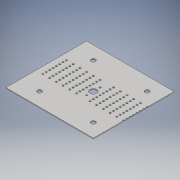
# Autodesk Inventor part: Drill Jig Base
Saved by Autodesk Inventor 2018 (Build 220112000, 112)
## iProperties
Created: 2018-12-05
Part Number: Drill Jig Base
Material: Generic
Document SubType Name: Modeling
Designer: gbgic
Density: 1 g/cm^3
Appearance: Default
Author: gbgic
Autodesk Inventor part; units mm, degrees
ref_plane "YZ Plane" through (0, 0, 0) normal (1, 0, 0) x (0, 1, 0)
ref_plane "XZ Plane" through (0, 0, 0) normal (0, 1, 0) x (-1, 0, 0)
ref_plane "XY Plane" through (0, 0, 0) normal (0, 0, 1) x (1, 0, 0)
sketch "Sketch1" plane through (0, 0, 0) normal (1, 0, 0) x (0, 1, 0)
  line L0 (4.9868, -9.3187) -> (4.9868, 295.4813)
  line L1 (4.9868, 295.4813) -> (-325.2132, 295.4813)
  line L2 (4.9868, -9.3187) -> (-325.2132, -9.3187)
  line L3 (-325.2132, 295.4813) -> (-325.2132, -9.3187)
  point P0 (0, 0)
  dimension "d73" = 330.2
  dimension "d74" = 330.2
  dimension "d75" = 304.8
  constraints: 8 end point, 2 horizontal, 1 vertical
  measures "d73" distance of L0.end L1.end
  measures "d74" distance of L0.start L2.end
  measures "d75" distance of L1.end L2.end
extrude "Extrusion1" add sketch "Sketch1" along normal blind 3.175
sketch "Sketch2" plane through (3.175, 0, 0) normal (1, 0, 0) x (0, 0, -1)
  line L0 (-143.0813, 4.9868) -> (-143.0813, -147.4132)
  circle A0 centre (-143.0813, -147.4132) radius 12.7
  point P0 (0, 0)
  point P1 (9.3187, 4.9868)
  dimension "d4" = 152.4
  dimension "d5" = 25.4
  constraints: 2 end point, 1 centre point, 1 coincident
  measures "d4" distance of L0.start L0.end
  measures "d5" diameter of A0
extrude "Extrusion2" cut sketch "Sketch2" against normal blind 50.8
sketch "Sketch3" plane through (3.175, 0, 0) normal (1, 0, 0) x (0, 0, -1)
  circle A0 centre (-143.0813, -147.4132) radius 12.7 projected
  circle A1 centre (-143.0813, -122.0132) radius 3.175
  circle A2 centre (-143.0813, -96.6132) radius 3.175
  circle A3 centre (-143.0813, -71.2132) radius 3.175
  circle A4 centre (-143.0813, -45.8132) radius 3.175
  circle A5 centre (-143.0813, -20.4132) radius 3.175
  circle A6 centre (-143.0813, 4.9868) radius 3.175
  line L0 (9.3187, -299.8132) -> (9.3187, 4.9868) projected
  circle A7 centre (-143.0813, -172.8132) radius 3.175
  circle A8 centre (-143.0813, -198.2132) radius 3.175
  circle A9 centre (-143.0813, -249.0132) radius 3.175
  circle A10 centre (-143.0813, -223.6132) radius 3.175
  circle A11 centre (-143.0813, -299.8132) radius 3.175
  circle A12 centre (-143.0813, -274.4132) radius 3.175
  circle A13 centre (-155.7813, -122.0132) radius 3.175
  circle A14 centre (-155.7813, -96.6132) radius 3.175
  circle A15 centre (-155.7813, -45.8132) radius 3.175
  circle A16 centre (-155.7813, -71.2132) radius 3.175
  circle A17 centre (-155.7813, 4.9868) radius 3.175
  circle A18 centre (-155.7813, -20.4132) radius 3.175
  circle A19 centre (-155.7813, -299.8132) radius 3.175
  circle A20 centre (-155.7813, -249.0132) radius 3.175
  circle A21 centre (-155.7813, -274.4132) radius 3.175
  circle A22 centre (-155.7813, -223.6132) radius 3.175
  circle A23 centre (-155.7813, -198.2132) radius 3.175
  circle A24 centre (-155.7813, -172.8132) radius 3.175
  line L1 (-155.7813, -299.8132) -> (-168.4813, -299.8132) construction
  line L2 (-168.4813, -299.8132) -> (-181.1813, -299.8132) construction
  line L3 (-181.1813, -299.8132) -> (-193.8813, -299.8132) construction
  line L4 (-143.0813, -299.8132) -> (-130.3813, -299.8132) construction
  line L5 (-130.3813, -299.8132) -> (-117.6813, -299.8132) construction
  line L6 (-117.6813, -299.8132) -> (-104.9813, -299.8132) construction
  circle A25 centre (-168.4813, -122.0132) radius 3.175
  circle A26 centre (-168.4813, -96.6132) radius 3.175
  circle A27 centre (-168.4813, -45.8132) radius 3.175
  circle A28 centre (-168.4813, -71.2132) radius 3.175
  circle A29 centre (-168.4813, 4.9868) radius 3.175
  circle A30 centre (-168.4813, -20.4132) radius 3.175
  circle A31 centre (-168.4813, -299.8132) radius 3.175
  circle A32 centre (-168.4813, -249.0132) radius 3.175
  circle A33 centre (-168.4813, -274.4132) radius 3.175
  circle A34 centre (-168.4813, -223.6132) radius 3.175
  circle A35 centre (-168.4813, -198.2132) radius 3.175
  circle A36 centre (-168.4813, -172.8132) radius 3.175
  circle A37 centre (-181.1813, -122.0132) radius 3.175
  circle A38 centre (-181.1813, -96.6132) radius 3.175
  circle A39 centre (-181.1813, -45.8132) radius 3.175
  circle A40 centre (-181.1813, -71.2132) radius 3.175
  circle A41 centre (-181.1813, 4.9868) radius 3.175
  circle A42 centre (-181.1813, -20.4132) radius 3.175
  circle A43 centre (-181.1813, -299.8132) radius 3.175
  circle A44 centre (-181.1813, -249.0132) radius 3.175
  circle A45 centre (-181.1813, -274.4132) radius 3.175
  circle A46 centre (-181.1813, -223.6132) radius 3.175
  circle A47 centre (-181.1813, -198.2132) radius 3.175
  circle A48 centre (-181.1813, -172.8132) radius 3.175
  circle A49 centre (-193.8813, -122.0132) radius 3.175
  circle A50 centre (-193.8813, -96.6132) radius 3.175
  circle A51 centre (-193.8813, -45.8132) radius 3.175
  circle A52 centre (-193.8813, -71.2132) radius 3.175
  circle A53 centre (-193.8813, 4.9868) radius 3.175
  circle A54 centre (-193.8813, -20.4132) radius 3.175
  circle A55 centre (-193.8813, -299.8132) radius 3.175
  circle A56 centre (-193.8813, -249.0132) radius 3.175
  circle A57 centre (-193.8813, -274.4132) radius 3.175
  circle A58 centre (-193.8813, -223.6132) radius 3.175
  circle A59 centre (-193.8813, -198.2132) radius 3.175
  circle A60 centre (-193.8813, -172.8132) radius 3.175
  circle A61 centre (-130.3813, -122.0132) radius 3.175
  circle A62 centre (-130.3813, -96.6132) radius 3.175
  circle A63 centre (-130.3813, -45.8132) radius 3.175
  circle A64 centre (-130.3813, -71.2132) radius 3.175
  circle A65 centre (-130.3813, 4.9868) radius 3.175
  circle A66 centre (-130.3813, -20.4132) radius 3.175
  circle A67 centre (-130.3813, -299.8132) radius 3.175
  circle A68 centre (-130.3813, -249.0132) radius 3.175
  circle A69 centre (-130.3813, -274.4132) radius 3.175
  circle A70 centre (-130.3813, -223.6132) radius 3.175
  circle A71 centre (-130.3813, -198.2132) radius 3.175
  circle A72 centre (-130.3813, -172.8132) radius 3.175
  line L7 (-117.6813, -299.8132) -> (-104.9813, -299.8132) construction
  circle A73 centre (-117.6813, -299.8132) radius 3.175
  circle A74 centre (-117.6813, -45.8132) radius 3.175
  circle A75 centre (-117.6813, -71.2132) radius 3.175
  circle A76 centre (-117.6813, -96.6132) radius 3.175
  circle A77 centre (-117.6813, -122.0132) radius 3.175
  circle A78 centre (-117.6813, 4.9868) radius 3.175
  circle A79 centre (-117.6813, -274.4132) radius 3.175
  circle A80 centre (-117.6813, -249.0132) radius 3.175
  circle A81 centre (-117.6813, -223.6132) radius 3.175
  circle A82 centre (-117.6813, -198.2132) radius 3.175
  circle A83 centre (-117.6813, -172.8132) radius 3.175
  circle A84 centre (-117.6813, -20.4132) radius 3.175
  line L8 (-104.9813, -299.8132) -> (-92.2813, -299.8132) construction
  circle A85 centre (-104.9813, -299.8132) radius 3.175
  circle A86 centre (-104.9813, -45.8132) radius 3.175
  circle A87 centre (-104.9813, -71.2132) radius 3.175
  circle A88 centre (-104.9813, -96.6132) radius 3.175
  circle A89 centre (-104.9813, -122.0132) radius 3.175
  circle A90 centre (-104.9813, 4.9868) radius 3.175
  circle A91 centre (-104.9813, -274.4132) radius 3.175
  circle A92 centre (-104.9813, -249.0132) radius 3.175
  circle A93 centre (-104.9813, -223.6132) radius 3.175
  circle A94 centre (-104.9813, -198.2132) radius 3.175
  circle A95 centre (-104.9813, -172.8132) radius 3.175
  circle A96 centre (-104.9813, -20.4132) radius 3.175
  point P0 (0, 0)
  dimension "d9" = 6.35
  dimension "d11" = 6.35
  dimension "d12" = 6.35
  dimension "d13" = 6.35
  dimension "d14" = 6.35
  dimension "d15" = 6.35
  dimension "d77" = 6.35
  dimension "d78" = 6.35
  dimension "d79" = 6.35
  dimension "d80" = 6.35
  dimension "d81" = 6.35
  dimension "d82" = 6.35
  dimension "d83" = 12.7
  dimension "d84" = 12.7
  dimension "d85" = 12.7
  dimension "d86" = 12.7
  dimension "d87" = 12.7
  dimension "d88" = 12.7
  dimension "d89" = 6.35
  dimension "d90" = 6.35
  dimension "d91" = 6.35
  dimension "d92" = 6.35
  dimension "d93" = 6.35
  dimension "d94" = 6.35
  dimension "d95" = 6.35
  dimension "d96" = 6.35
  dimension "d97" = 6.35
  dimension "d98" = 6.35
  dimension "d99" = 6.35
  dimension "d100" = 6.35
  dimension "d101" = 6.35
  dimension "d102" = 6.35
  dimension "d103" = 6.35
  dimension "d104" = 6.35
  dimension "d105" = 6.35
  dimension "d106" = 6.35
  dimension "d107" = 6.35
  dimension "d108" = 6.35
  dimension "d109" = 6.35
  dimension "d110" = 6.35
  dimension "d111" = 6.35
  dimension "d112" = 6.35
  dimension "d113" = 12.7
  dimension "d114" = 6.35
  dimension "d115" = 6.35
  dimension "d116" = 6.35
  dimension "d117" = 6.35
  dimension "d118" = 6.35
  dimension "d119" = 6.35
  dimension "d120" = 12.7
  dimension "d121" = 6.35
  dimension "d122" = 6.35
  dimension "d123" = 6.35
  dimension "d124" = 6.35
  dimension "d125" = 6.35
  dimension "d126" = 6.35
  constraints: 96 centre point, 16 end point, 5 horizontal, 3 point on line
  measures "d9" diameter of A1
  measures "d11" diameter of A2
  measures "d12" diameter of A3
  measures "d13" diameter of A4
  measures "d14" diameter of A5
  measures "d15" diameter of A6
  measures "d77" diameter of A13
  measures "d78" diameter of A14
  measures "d79" diameter of A16
  measures "d80" diameter of A15
  measures "d81" diameter of A18
  measures "d82" diameter of A17
  measures "d83" distance of L1.start L1.end
  measures "d84" distance of L1.end L2.end
  measures "d85" distance of L2.end L3.end
  measures "d86" distance of L4.start L4.end
  measures "d87" distance of L5.end L4.end
  measures "d88" distance of L5.end L6.end
  measures "d89" diameter of A25
  measures "d90" diameter of A26
  measures "d91" diameter of A28
  measures "d92" diameter of A27
  measures "d93" diameter of A30
  measures "d94" diameter of A29
  measures "d95" diameter of A37
  measures "d96" diameter of A38
  measures "d97" diameter of A40
  measures "d98" diameter of A39
  measures "d99" diameter of A42
  measures "d100" diameter of A41
  measures "d101" diameter of A49
  measures "d102" diameter of A50
  measures "d103" diameter of A52
  measures "d104" diameter of A51
  measures "d105" diameter of A54
  measures "d106" diameter of A53
  measures "d107" diameter of A61
  measures "d108" diameter of A62
  measures "d109" diameter of A64
  measures "d110" diameter of A63
  measures "d111" diameter of A66
  measures "d112" diameter of A65
  measures "d113" distance of L5.end L7.end
  measures "d114" diameter of A77
  measures "d115" diameter of A76
  measures "d116" diameter of A75
  measures "d117" diameter of A74
  measures "d118" diameter of A84
  measures "d119" diameter of A78
  measures "d120" distance of L8.start L8.end
  measures "d121" diameter of A89
  measures "d122" diameter of A88
  measures "d123" diameter of A87
  measures "d124" diameter of A86
  measures "d125" diameter of A96
  measures "d126" diameter of A90
sketch "Sketch4" plane through (3.175, 0, 0) normal (1, 0, 0) x (0, 0, -1)
  circle A0 centre (-143.0813, -147.4132) radius 12.7 projected
  circle A1 centre (-117.6813, -147.4132) radius 3.175
  line L0 (-143.0813, -147.4132) -> (-155.7813, -147.4132) construction
  line L1 (-155.7813, -147.4132) -> (-168.4813, -147.4132) construction
  circle A2 centre (-168.4813, -147.4132) radius 3.175
  point P0 (0, 0)
  dimension "d56" = 6.35
  dimension "d127" = 12.7
  dimension "d128" = 12.7
  dimension "d130" = 6.35
  constraints: 4 end point, 2 centre point, 1 coincident, 1 horizontal, 1 point on line
  measures "d56" diameter of A1
  measures "d127" distance of L0.start L0.end
  measures "d128" distance of L0.end L1.end
  measures "d130" diameter of A2
sketch "Sketch5" plane through (3.175, 0, 0) normal (1, 0, 0) x (0, 0, -1)
  line L0 (-295.4813, 4.9868) -> (-295.4813, -299.8132) projected
  circle A0 centre (-244.6813, -249.0132) radius 7.9375
  circle A1 centre (-41.4813, -249.0132) radius 7.9375
  line L1 (-244.6813, -249.0132) -> (-244.6813, -45.8132) construction
  circle A2 centre (-244.6813, -45.8132) radius 7.9375
  circle A3 centre (-41.4813, -45.8132) radius 7.9375
  point P0 (0, 0)
  dimension "d63" = 15.875
  dimension "d67" = 203.2
  dimension "d69" = 15.875
  dimension "d70" = 15.875
  constraints: 4 centre point, 2 end point, 1 coincident, 1 vertical
  measures "d63" diameter of A0
  measures "d67" distance of L1.start L1.end
  measures "d69" diameter of A2
  measures "d70" diameter of A3
extrude "Extrusion5" cut sketch "Sketch5" against normal blind 914.4
extrude "Extrusion6" cut sketch "Sketch3" against normal blind 76.2 contours A1 | A2 | A3 | A4 | A5 | A6 | A7 | A8 | A9 | A10 | A11 | A12 | A13 | A14 | A15 | A16 | A17 | A18 | A19 | A20 | A21 | A22 | A23 | A24 | A25 | A26 | A27 | A28 | A29 | A30 | A31 | A32 | A33 | A34 | A35 | A36 | A37 | A38 | A39 | A40 | A41 | A42 | A43 | A44 | A45 | A46 | A47 | A48 | A49 | A50 | A51 | A52 | A53 | A54 | A55 | A56 | A57 | A58 | A59 | A60 | A61 | A62 | A63 | A64 | A65 | A66 | A67 | A68 | A69 | A70 | A71 | A72 | A73 | A74 | A75 | A76 | A77 | A78 | A79 | A80 | A81 | A82 | A83 | A84 | A85 | A86 | A87 | A88 | A89 | A90 | A91 | A92 | A93 | A94 | A95 | A96
extrude "Extrusion8" cut sketch "Sketch4" against normal blind 76.2
body "Solid1"
